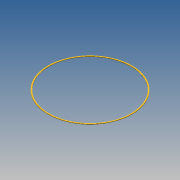
# Autodesk Inventor part: hubGuideRingOuter
Saved by Autodesk Inventor 2014 SP1 (Build 180222100, 222)
## iProperties
Created: 2014-12-05
Part Number: hubGuideRingOuter
Material: Gold
Document SubType Name: Modeling
Designer: Dave
Density: 19.3 g/cm^3
Appearance: Gold - Metal
Mass: 900.443 g
Surface Area: 514.308 cm^2
Volume: 46.6551 cm^3
Author: Dave
Autodesk Inventor part; units mm, degrees
ref_plane "YZ Plane" through (0, 0, 0) normal (1, 0, 0) x (0, 1, 0)
ref_plane "XZ Plane" through (0, 0, 0) normal (0, 1, 0) x (-1, 0, 0)
ref_plane "XY Plane" through (0, 0, 0) normal (0, 0, 1) x (1, 0, 0)
sketch "Sketch1" plane through (0, 0, 0) normal (0, 1, 0) x (-1, 0, 0)
  circle A0 centre (0, 0) radius 228.6
  circle A1 centre (0, 0) radius 234.95
  dimension "d0" = 457.2
  dimension "d1" = 6.35
  constraints: 2 centre point, 1 coincident
  measures "d0" diameter of A0
  measures "d1" radial gap between concentric circles of A0 A1
extrude "Extrusion1" add sketch "Sketch1" along normal blind 2.54
equation "\"d0\" = hubInnerDiam"
equation "\"hubOuterDiam\" = 914.4"
equation "\"hubInnerDiam\" = 0.5 * hubOuterDiam"
body "Solid1"
